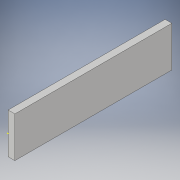
# Autodesk Inventor part: MotorPlate
Saved by Autodesk Inventor 2017 (Build 210142000, 142)
## iProperties
Created: 2017-10-13
Part Number: MotorPlate
Material: Generic
Document SubType Name: Modeling
Designer: Kenneth
Density: 1 g/cm^3
Appearance: Default
Author: Kenneth
Autodesk Inventor part; units mm, degrees
ref_plane "YZ Plane" through (0, 0, 0) normal (1, 0, 0) x (0, 1, 0)
ref_plane "XZ Plane" through (0, 0, 0) normal (0, 1, 0) x (-1, 0, 0)
ref_plane "XY Plane" through (0, 0, 0) normal (0, 0, 1) x (1, 0, 0)
sketch "Sketch1" plane through (0, 0, 0) normal (1, 0, 0) x (0, 1, 0)
  line L0 (-38.1, 147.8788) -> (38.1, 147.8788)
  line L1 (38.1, 147.8788) -> (38.1, -147.8788)
  line L2 (38.1, -147.8788) -> (-38.1, -147.8788)
  line L3 (-38.1, -147.8788) -> (-38.1, 147.8788)
  line L4 (-38.1, 147.8788) -> (38.1, -147.8788) construction
  line L5 (38.1, 147.8788) -> (-38.1, -147.8788) construction
  point P0 (0, 0)
  dimension "d0" = 295.7576
  dimension "d1" = 76.2
  constraints: 12 end point, 2 midpoint, 2 parallel, 1 horizontal, 1 perpendicular
  measures "d0" distance of L0.end L1.end
  measures "d1" distance of L0.start L0.end
extrude "Extrusion1" add sketch "Sketch1" along normal blind 12.7
sketch "Sketch2" plane through (0, -38.1, 147.8788) normal (0, 0, 1) x (1, 0, 0)
  point P0 (0, 38.1)
body "Solid1"
